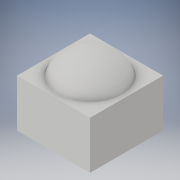
# Autodesk Inventor part: mouse ball
Saved by Autodesk Inventor 2017 (Build 210142000, 142)
## iProperties
Created: 2018-03-13
Part Number: mouse ball
Material: Generic
Document SubType Name: Modeling
Designer: Braxton
Density: 1 g/cm^3
Appearance: Default
Author: Braxton
Autodesk Inventor part; units mm, degrees
ref_plane "YZ Plane" through (0, 0, 0) normal (1, 0, 0) x (0, 1, 0)
ref_plane "XZ Plane" through (0, 0, 0) normal (0, 1, 0) x (-1, 0, 0)
ref_plane "XY Plane" through (0, 0, 0) normal (0, 0, 1) x (1, 0, 0)
sketch "Sketch1" plane through (0, 0, 0) normal (1, 0, 0) x (0, 1, 0)
  arc A0 (38.9763, 0) -> (-38.9763, 0) centre (0, 0) ccw
  arc A1 (42.4307, 0) -> (-42.4307, 0) centre (0, 0) ccw
  line L0 (-45.8851, 0) -> (-45.8851, 45.8851)
  line L1 (13.8845, 45.8851) -> (-45.8851, 45.8851)
  line L2 (13.8845, 45.8851) -> (13.8845, 0)
  line L3 (-45.8851, 0) -> (-45.8851, -45.8851)
  line L4 (13.8845, -45.8851) -> (-45.8851, -45.8851)
  line L5 (13.8845, -45.8851) -> (13.8845, 0)
  line L6 (42.9387, 0) -> (42.4307, 0)
  line L7 (38.9763, 0) -> (42.4307, 0)
  line L8 (38.9763, 0) -> (-38.9763, 0)
  line L9 (-38.9763, 0) -> (-42.4307, 0)
  line L10 (-42.4307, 0) -> (-42.9387, 0)
  dimension "d0" = 77.9526
  dimension "d3" = 45.8851
  dimension "d4" = 45.8851
  dimension "d10" = 3.4544
  dimension "d19" = 91.7702
  constraints: 22 end point, 4 point on circle, 3 collinear, 2 centre point, 2 coincident, 2 perpendicular, 1 horizontal, 1 other
  measures "d0" diameter of A0
  measures "d3" distance from line of A1.centre L1
  measures "d4" distance from line of L0 A1.centre
  measures "d10" radial gap between concentric circles of A0 A1
  measures "d19" distance between parallel lines of L4 L1
extrude "cube to cut from" add sketch "Sketch1" along normal mid plane 91.7702 contours L2 L8 A0 | A0 L9 A1 L2 | L5 L4 L3 L0 L1 L2 A1 L9 L8 picked at (-21.0569, 2.7719)
sketch "Sketch2" plane through (0, 0, 0) normal (1, 0, 0) x (0, 1, 0)
  arc A0 (42.9387, 0) -> (-42.9387, 0) centre (0, 0) ccw
  line L0 (42.9387, 0) -> (-42.9387, 0)
  dimension "d17" = 85.8774
  constraints: 2 end point, 2 point on circle, 1 centre point, 1 coincident, 1 horizontal
  measures "d17" diameter of A0
revolve "cut out for mouse ball" cut sketch "Sketch2" angle 360 about axis through (0, 42.9387, 0) along (0, -1, 0)
revolve "mouse ball" add sketch "Sketch1" angle 360 about axis through (0, 38.9763, 0) along (0, -1, 0) separate body contours A0 L2 A1 L7 | A0 L9 A1 L2
equation "\"d3\" = 0.5 * d0 + 2 * d1"
equation "\"d4\" = 0.5 * d0 + 2 * d1"
equation "\"d8\" = d19"
equation "\"d17\" = 2 * d10 + d0 + 2 * d11"
equation "\"d1\" = 3.4544"
equation "\"d11\" = 0.508"
